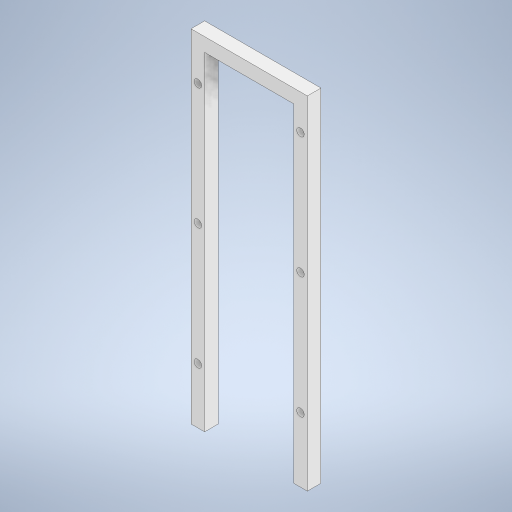
# Autodesk Inventor part: Sustentação Trilhos fixos
Saved by Autodesk Inventor 2024 (Build 280153000, 153)
## iProperties
Created: 2023-05-11
Part Number: Sustentação Trilhos fixos
Material: Plástico PET
Document SubType Name: Modeling
Designer: jpjoa
Density: 1.541 g/cm^3
Appearance: Branco
Author: jpjoa
Autodesk Inventor part; units mm, degrees
ref_plane "YZ Plane" through (0, 0, 0) normal (1, 0, 0) x (0, 1, 0)
ref_plane "XZ Plane" through (0, 0, 0) normal (0, 1, 0) x (-1, 0, 0)
ref_plane "XY Plane" through (0, 0, 0) normal (0, 0, 1) x (1, 0, 0)
sketch "Esboço1" plane through (0, 0, 0) normal (0, 1, 0) x (-1, 0, 0)
  line L0 (0, 0) -> (0, -5.4)
  line L1 (0, -5.4) -> (5.4, -5.4)
  line L2 (5.4, -5.4) -> (5.4, 0)
  line L3 (5.4, 0) -> (0, 0)
  line L4 (40.622, 0) -> (40.622, -5.4)
  line L5 (40.622, -5.4) -> (46.022, -5.4)
  line L6 (46.022, -5.4) -> (46.022, 0)
  line L7 (46.022, 0) -> (40.622, 0)
  line L8 (40.622, 0) -> (5.4, 0)
  line L9 (5.4, -5.4) -> (40.622, -5.4)
  point P0 (0, -2.7)
  point P1 (5.4, -2.7)
  point P2 (40.622, -2.7)
  point P3 (46.022, -2.7)
  point P4 (43.322, -5.4)
  point P5 (2.7, -5.4)
  point P6 (43.322, 0)
  point P7 (2.7, 0)
  point P8 (0, 0)
  dimension "d29" = 35.222
  dimension "d30" = 5.4
  constraints: 20 end point, 8 midpoint, 6 perpendicular, 2 coincident, 2 equal length, 2 horizontal alignment, 2 vertical, 1 collinear, 1 horizontal
  measures "d29" distance between parallel lines of L2 L4
  measures "d30" distance of L4.end L5.end
extrude "Extrusão1" add sketch "Esboço1" against normal blind 130 contours L3 L2 L1 L0 | L7 L6 L5 L4
extrude "Extrusão4" add sketch "Esboço1" along normal blind 5.4
sketch "Esboço5" plane through (-40.622, 0, 0) normal (0, 0, 1) x (1, 0, 0)
  circle A0 centre (37.922, -104.396) radius 1.5
  circle A1 centre (37.922, -56.396) radius 1.5
  circle A2 centre (37.922, -8.397) radius 1.5
  circle A3 centre (-2.7, -107.95) radius 1.5
  circle A4 centre (-2.7, -59.95) radius 1.5
  circle A5 centre (-2.7, -11.951) radius 1.5
  line L0 (40.622, -130) -> (35.222, -130) projected
  line L1 (0, -130) -> (-5.4, -130) projected
  line L2 (37.7913, -105.8903) -> (103.7232, -105.8903) construction
  line L3 (38.0527, -57.8903) -> (-2.5693, -61.4443)
  line L4 (38.0527, -9.8913) -> (-2.5693, -13.4453)
  line L5 (-2.5693, -109.4443) -> (38.0527, -105.8903)
  point P0 (40.622, 0)
  point P1 (37.922, -130)
  point P2 (-2.7, -130)
  dimension "d33" = 3
  dimension "d34" = 3
  dimension "d36" = 3
  dimension "d38" = 3
  dimension "d40" = 3
  dimension "d42" = 3
  dimension "d44" = 25.604
  dimension "d45" = 48
  dimension "d46" = 47.999
  dimension "d52" = 5
  constraints: 8 end point, 6 vertical alignment, 2 midpoint, 2 parallel, 1 horizontal, 1 point on line, 24 other
  measures "d44" distance from line of L0 point (37.922, -104.396)
  measures "d45" distance of point (37.922, -104.396) point (37.922, -56.396)
  measures "d46" distance of point (37.922, -56.396) point (37.922, -8.397)
  measures "d52" angle of L1 L5
extrude "Extrusão5" cut sketch "Esboço5" against normal through all
equation "\"d29\" = Largura_trilhos"
equation "\"d33\" = Parafuso"
equation "\"d34\" = d35"
equation "\"d36\" = d37"
equation "\"d38\" = d39"
equation "\"d40\" = d41"
equation "\"d42\" = d43"
equation "\"Largura_trilhos\" = 35.222"
equation "\"Parafuso\" = 3"
equation "\"d11\" = 3"
equation "\"d13\" = 3"
equation "\"d15\" = 3"
equation "\"d17\" = 3"
equation "\"d19\" = 3"
equation "\"d35\" = 3"
equation "\"d37\" = 3"
equation "\"d39\" = 3"
equation "\"d41\" = 3"
equation "\"d43\" = 3"
